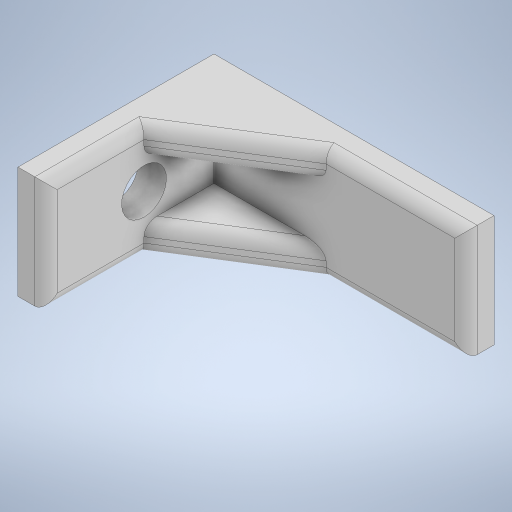
# Autodesk Inventor part: Part1
Saved by Autodesk Inventor 2024.2 (Build 282272000, 272)
## iProperties
Created: 2024-04-19
Part Number: Part1
Material: Generic
Document SubType Name: Modeling
Designer: jebes windows
Density: 1 g/cm^3
Appearance: Default
Author: jebes windows
Autodesk Inventor part; units mm, degrees
ref_plane "YZ Plane" through (0, 0, 0) normal (1, 0, 0) x (0, 1, 0)
ref_plane "XZ Plane" through (0, 0, 0) normal (0, 1, 0) x (-1, 0, 0)
ref_plane "XY Plane" through (0, 0, 0) normal (0, 0, 1) x (1, 0, 0)
sketch "Sketch1" plane through (0, 0, 0) normal (0, 1, 0) x (-1, 0, 0)
  line L0 (25, 10) -> (-25, 10)
  line L1 (-25, 10) -> (-25, -10)
  line L2 (-25, -10) -> (25, -10)
  line L3 (25, -10) -> (25, 10)
  line L4 (25, 10) -> (-25, -10) construction
  line L5 (-25, 10) -> (25, -10) construction
  point P0 (0, 0)
  dimension "d0" = 50
  dimension "d1" = 20
  constraints: 12 end point, 2 midpoint, 2 parallel, 1 horizontal, 1 perpendicular
  measures "d0" distance of L2.end L1.end
  measures "d1" distance of L1.end L0.end
extrude "Extrusion1" add sketch "Sketch1" along normal blind 5
sketch "Sketch2" plane through (0, 0, 0) normal (0, -1, 0) x (1, 0, 0)
  line L0 (-25, -10) -> (-25, 10) projected
  line L1 (-25, 10) -> (-20, 10)
  line L2 (-25, 10) -> (25, 10) projected
  line L3 (-20, 10) -> (-20, -10)
  line L4 (25, -10) -> (-25, -10) projected
  line L5 (-25, -10) -> (-20, -10)
  line L6 (-25, 10) -> (-25, -10)
  point P0 (0, 0)
  dimension "d4" = 5
  constraints: 8 end point, 2 collinear, 1 perpendicular, 1 point on line
  measures "d4" distance of L0.end L1.end
extrude "Extrusion2" add sketch "Sketch2" along normal blind 30
sketch "Sketch3" plane through (-20, 0, 10) normal (1, 0, 0) x (0, 0, -1)
  point P0 (10, 0)
sketch "Sketch4" plane through (-25, 5, 10) normal (0, 0, 1) x (1, 0, 0)
  line L0 (5, -5) -> (50, -5) projected
  line L1 (50, -5) -> (50, 0) projected
  line L2 (0, 0) -> (50, 0) projected
  line L3 (0, -35) -> (0, 0) projected
  line L4 (5, -35) -> (0, -35) projected
  line L5 (5, -5) -> (5, -35) projected
  line L6 (25, -5) -> (5, -17.5)
  dimension "d7" = 10.6
  constraints: 2 end point, 1 point on line
  measures "d7" distance from line of L0.start L6
extrude "Extrusion3" add sketch "Sketch4" against normal blind 5 contours L0 L6 L5
mirror "Mirror1" about plane through (0, 0, 0) normal (0, 0, 1) of "Extrusion3"
sketch "Sketch5" plane through (-20, -30, 10) normal (1, 0, 0) x (0, 0, -1)
  circle A0 centre (10, 17.5) radius 4
  line L0 (0, 30) -> (20, 30) projected
  line L1 (0, 17.5) -> (0, 0) projected
  point P0 (10, 30)
  point P1 (10, 30)
  dimension "d10" = 8
  dimension "d11" = 12.5
  dimension "d12" = 10
  constraints: 1 centre point, 1 midpoint
  measures "d10" diameter of A0
  measures "d11" distance of point (10, 30) A0.centre
  measures "d12" distance from line of L1 A0.centre
extrude "Extrusion4" cut sketch "Sketch5" against normal blind 5
fillet "Fillet1" radius 2 2 edges at (-10, -6.25, 5) (-10, -6.25, -5)
fillet "Fillet2" radius 2 8 edges at (12.5, 0, -10) (-10, -6.25, -10) (25, 0, 0) (12.5, 0, 10) (-10, -6.25, 10) (-20, -21.25, -10) (-20, -30, 0) (-20, -21.25, 10)
body "Solid1"
